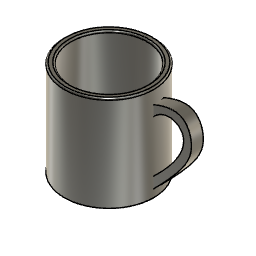
cup v1 (Autodesk Fusion 360 design; units mm, degrees)
Autodesk Fusion 360 part; units mm, degrees
sketch "Sketch1" plane through (0, 0, 0) normal (0, 0, 1) x (1, 0, 0)
sketch "Sketch2" plane through (0, 0, 0) normal (0, 0, 1) x (1, 0, 0)
  circle A0 centre (0, 120) radius 37.5
  dimension "d2" = 75
  measures "d2" diameter of A0
extrude "Extrude1" add sketch "Sketch2" along normal blind 80 makes body 1
sketch "Sketch3" plane through (0, 0, 80) normal (0, 0, 1) x (-1, 0, 0)
  circle A0 centre (0, -120) radius 37.5
  circle A1 centre (0, -120) radius 32.0974
  constraint concentric A0 A1
extrude "Extrude2" cut sketch "Sketch3" against normal blind 75 contours A1 bodies 1
fillet "Fillet1" radius 1.3 2 edges at (29.9253, 108.3931, 80) (-34.9623, 106.4394, 80) on bodies 1
sketch "Sketch4" plane through (0, 0, 0) normal (0, 1, 0) x (1, 0, 0)
  spline S0 degree 5 poles (37.0112, -57.3867) (37.7017, -58.1498) (39.0971, -59.5816) (41.2335, -61.4456) (44.1689, -63.3597) (47.963, -64.7782) (51.8117, -65.2003) (55.5719, -64.6159) (58.9874, -63.0463) (61.7351, -60.5383) (63.4909, -57.1519) (63.9948, -52.9546) (63.1099, -48.0158) (60.7806, -42.401) (57.0063, -36.1667) (51.8166, -29.3584) (46.5642, -23.4782) (42.0209, -18.8325) (38.7255, -15.6315) (37.0112, -14.005) knots 0 0 0 0 0 0 0.066667 0.133333 0.2 0.266667 0.333333 0.4 0.466667 0.533333 0.6 0.666667 0.733333 0.8 0.866667 0.933333 1 1 1 1 1 1
  spline S1 degree 5 poles (37.0112, -57.3867) (37.0112, -57.7625) (37.0112, -58.514) (37.0112, -59.6412) (37.0112, -61.1442) (37.0112, -63.0229) (37.0112, -64.5259) (37.0112, -65.6532) (37.0112, -66.4047) (37.0112, -66.7804) knots 0 0 0 0 0 0 0.2 0.4 0.6 0.8 1 1 1 1 1 1
  spline S2 degree 5 poles (37.0112, -66.7804) (38.6955, -67.5099) (41.9503, -68.8276) (46.4913, -70.3803) (51.8612, -71.5999) (57.4274, -71.7125) (61.8654, -70.47) (65.2291, -68.0103) (67.6405, -64.6018) (69.2887, -60.6613) (70.2073, -56.439) (70.3854, -52.1122) (69.7911, -47.7774) (68.4408, -43.4829) (66.4088, -39.2394) (63.7997, -35.0327) (60.7306, -30.8344) (57.312, -26.6131) (53.6265, -22.3462) (49.7299, -18.02) (45.6573, -13.6272) (42.2736, -10.0571) (39.6685, -7.3481) (37.9019, -5.5281) (37.0112, -4.6146) knots 0 0 0 0 0 0 0.05 0.1 0.15 0.2 0.25 0.3 0.35 0.4 0.45 0.5 0.55 0.6 0.65 0.7 0.75 0.8 0.85 0.9 0.95 1 1 1 1 1 1
  spline S3 degree 5 poles (37.0112, -4.6146) (37.0112, -4.9902) (37.0112, -5.7415) (37.0112, -6.8683) (37.0112, -8.3708) (37.0112, -10.2489) (37.0112, -11.7513) (37.0112, -12.8782) (37.0112, -13.6294) (37.0112, -14.005) knots 0 0 0 0 0 0 0.2 0.4 0.6 0.8 1 1 1 1 1 1
  line L0 (61.6133, -72.0609) -> (70.2359, -61.4094)
  point P0 (52.6286, -64.9062)
  point P1 (63.0402, -57.3867)
  point P2 (65.9246, -66.7352)
  point P3 (70, -50)
  point P4 (60, -30)
  constraint midpoint P2 L0
extrude "Extrude3" add sketch "Sketch4" along normal blind 10 separate body makes body 2
move_body "Move1" bodies 2 to x (1, 0, 0) y (0, 1, 0) z (0, 0, 1) at (-0.939, 120, 0.3438)
